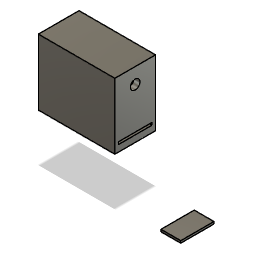
Kamera_arm-neu (Autodesk Fusion 360 design; units mm, degrees)
Autodesk Fusion 360 part; units mm, degrees
note: some values were not read from the file. Chosen so that the rebuilt part matches the saved one: which bodies a step acts on; which face or edge a step refers to. Set by a fixed rule: which sketch regions a step uses.
sketch "Skizze1" plane through (0, 0, 0) normal (0, 0, 1) x (1, 0, 0)
  line L0 (0, 0) -> (12, 0)
  line L1 (12, 0) -> (12, 24)
  line L2 (12, 24) -> (0, 24)
  line L3 (0, 24) -> (0, 0)
  dimension "d1" = 12
  dimension "d2" = 24
  constraint coincident L0.start L3.end
  constraint horizontal L0
  constraint perpendicular L0 L1
  constraint perpendicular L1 L2
  constraint perpendicular L0 L3
  measures "d1" distance of L0.start L0.end
  measures "d2" distance of L0.end L1.end
extrude "Extrusion1" add sketch "Skizze1" along normal blind 23 makes body 1
sketch "Skizze2" plane through (0, 0, 0) normal (0, 1, 0) x (1, 0, 0)
  line L0 (5, 5) -> (0.75, 5)
  circle A0 centre (2, 10.9) radius 1.5
  line L1 (0, 5.75) -> (0, 10)
  line L2 (0, 10) -> (0.8, 10)
  line L3 (0.8, 10) -> (0.8, 11.8)
  line L4 (0, 11.8) -> (0.8, 11.8)
  line L5 (0, 11.8) -> (0, 16.05)
  line L6 (0.75, 16.8) -> (5, 16.8)
  line L7 (5, 16.8) -> (5, 5)
  arc A1 (0, 5.75) -> (0.75, 5) centre (0.75, 5.75) ccw
  arc A2 (0.75, 16.8) -> (0, 16.05) centre (0.75, 16.05) ccw
  point P0 (0, 16.8)
  dimension "d7" = 3
  dimension "d9" = 5
  dimension "d10" = 0.75
  dimension "d11" = 0.75
  constraint horizontal L0
  constraint perpendicular L0 L1
  constraint coincident A0 L2.end
  constraint perpendicular L1 L2
  constraint coincident A0 L3.end
  constraint perpendicular L2 L3
  constraint perpendicular L3 L4
  constraint perpendicular L4 L5
  constraint perpendicular L5 L6
  constraint perpendicular L0 L7
  constraint tangent L0 A1
  constraint tangent L1 A1
  constraint coincident P0 L5
  constraint coincident P0 L6
  constraint tangent L5 A2
  constraint tangent L6 A2
  measures "d7" diameter of A0
  measures "d9" distance of L4.start P0
  measures "d10" radius of A1
  measures "d11" radius of A2
extrude "Extrusion2" add sketch "Skizze2" along normal blind 2.45 separate body contours L0 A0 L1 L2 L4 L5 L6 L7 A1 A2 makes body 2
move_body "Verschieben1" bodies 2 to x (1, 0, 0) y (0, 1, 0) z (0, 0, 1) at (0, 17.3532, -0.1472)
move_body "Verschieben2" bodies 2 to x (0, 0, 1) y (0, 1, 0) z (-1, 0, 0) at (-4.9472, 0, -4.9472)
copy_body "Körper kopieren/einfügen1" bodies 2 makes body 3
move_body "Verschieben3" bodies 3 to x (-1, 0, 0) y (0, 1, 0) z (0, 0, -1) at (12.15, 0, 25.1056)
move_body "Verschieben4" bodies 3 to x (1, 0, 0) y (0, 1, 0) z (0, 0, 1) at (0, 0, -2)
sketch "Skizze3" plane through (0, 0, 0) normal (0, 1, 0) x (1, 0, 0)
  circle A0 centre (25, -5) radius 6
  circle A1 centre (20, 9) radius 2.5
  circle A2 centre (31, -5) radius 2.75
  dimension "d14" = 12
  dimension "d15" = 5
  dimension "d16" = 5.5
  constraint coincident A0 A2.centre
  measures "d14" diameter of A0
  measures "d15" diameter of A1
  measures "d16" diameter of A2
extrude "Extrusion3" add sketch "Skizze3" along normal blind 2.5 separate body makes body 4 at (26.7719, 0, 5.8661) makes body 5 at (22.4969, 1.6667, -8.8754)
extrude "Extrusion4" add 1 faces at (26.6198, 2.5, 6.1216) along direction (0, 1, 0) blind 1.5 on bodies 4 bodies 4
move_body "Verschieben5" bodies 4 to x (1, 0, 0) y (0, 1, 0) z (0, 0, 1) at (0, 24, 0)
move_body "Verschieben6" bodies 4 to x (0, 0, 1) y (0, 1, 0) z (-1, 0, 0) at (10.9668, 0, -18.9668)
move_body "Verschieben7" bodies 5 to x (1, 0, 0) y (0, 1, 0) z (0, 0, 1) at (0, 28, 0)
move_body "Verschieben8" bodies 5 to x (1, 0, 0) y (0, 1, 0) z (0, 0, 1) at (-14, 0, 15)
combine "Kombinieren1" operation add target body 1 tool bodies 4
combine "Kombinieren2" operation add target body 5 tool bodies 1
combine "Kombinieren3" operation add target body 3 tool bodies 5 makes body 6 at (0, 8, 9.888)
combine "Kombinieren4" operation add target body 2 tool bodies 6
combine "Kombinieren5" operation add target body 2 tool bodies 3 makes body 7 at (10.468, 19.8032, 25.3466)
combine "Kombinieren6" operation add target body 7 tool bodies 2 makes body 8 at (0, 8, 9.888)
move_body "Verschieben9" bodies 7 to x (1, 0, 0) y (0, 1, 0) z (0, 0, 1) at (0, 0, -0.05)
move_body "Verschieben10" bodies 7 to x (1, 0, 0) y (0, 1, 0) z (0, 0, 1) at (0, 0, -0.05)
combine "Kombinieren7" operation add target body 7 tool bodies 8
move_body "Verschieben11" bodies 7 to x (1, 0, 0) y (0, 1, 0) z (0, 0, 1) at (0, 0, -28)
sketch "Skizze4" plane through (0, 0, 0) normal (0, 0, 1) x (1, 0, 0)
move_body "Verschieben12" bodies 7 to x (0, 0, -1) y (0, -1, 0) z (-1, 0, 0) at (0.1534, 30.5433, -0.1778)
sketch "Skizze5" plane through (0, 0, 0) normal (0, 0, 1) x (1, 0, 0)
  line L0 (55, 25) -> (105, 25)
  line L1 (105, 25) -> (105, 15)
  line L2 (55, -10) -> (55, 25)
  line L3 (55, -10) -> (105, 15)
  dimension "d21" = 50
  constraint horizontal L0
  constraint perpendicular L0 L1
  constraint perpendicular L0 L2
  measures "d21" distance of L0.start L0.end
extrude "Extrusion5" add sketch "Skizze5" along normal blind 20 separate body makes body 9
sketch "Skizze6" plane through (0, 0, 0) normal (0, 1, 0) x (1, 0, 0)
  circle A0 centre (125, -10) radius 2.5
  dimension "d24" = 5
  measures "d24" diameter of A0
hole "Bohrung1" at (95.1516, 25, 10.0122) direction (0, -1, 0) diameter 5 depth 2 tip angle 180 bodies 9
move_body "Verschieben13" bodies 9 to x (1, 0, 0) y (0, 1, 0) z (0, 0, 1) at (0, 0, -20)
sketch "Skizze7" plane through (0, 0, 0) normal (0, 0, 1) x (1, 0, 0)
  line L0 (125, 0) -> (131, 0)
  line L1 (131, 0) -> (131, 2.45)
  line L2 (164, 2.45) -> (164, 0)
  line L3 (164, 0) -> (170, 0)
  line L4 (170, 0) -> (170, 50)
  line L5 (170, 50) -> (125, 50)
  line L6 (125, 50) -> (125, 0)
  line L7 (131, 2.45) -> (136, 2.45)
  line L8 (136, 2.45) -> (136, 19.8)
  line L9 (164, 2.45) -> (159, 2.45)
  line L10 (159, 2.45) -> (159, 19.8)
  line L11 (136, 19.8) -> (159, 19.8)
  dimension "d31" = 2.45
  constraint horizontal L0
  constraint perpendicular L0 L1
  constraint perpendicular L2 L3
  constraint perpendicular L3 L4
  constraint perpendicular L4 L5
  constraint perpendicular L0 L6
  constraint perpendicular L1 L7
  constraint perpendicular L7 L8
  constraint perpendicular L2 L9
  constraint perpendicular L9 L10
  constraint perpendicular L10 L11
  measures "d31" distance of L0.end L1.end
extrude "Extrusion7" add sketch "Skizze7" against normal blind 30 separate body makes body 10
sketch "Skizze8" plane through (0, 0, 0) normal (0, 1, 0) x (1, 0, 0)
  line L0 (125, 40) -> (125, 49)
  line L1 (125, 49) -> (170, 49)
  line L2 (170, 49) -> (170, 40)
  line L3 (170, 40) -> (125, 40)
  line L4 (125, 55) -> (125, 64)
  line L5 (125, 64) -> (170, 64)
  line L6 (170, 64) -> (170, 55)
  line L7 (170, 55) -> (125, 55)
  constraint vertical L0
  constraint perpendicular L0 L1
  constraint perpendicular L1 L2
  constraint perpendicular L0 L3
  constraint perpendicular L1 L4
  constraint perpendicular L4 L5
  constraint perpendicular L1 L6
  constraint perpendicular L4 L7
extrude "Extrusion8" add sketch "Skizze8" along normal blind 20 separate body makes body 11 at (140, 13.3333, -49) makes body 12 at (140, 13.3333, -64)
move_body "Verschieben14" bodies 12 to x (1, 0, 0) y (0, 1, 0) z (0, 0, 1) at (0, 0, 55)
combine "Kombinieren8" operation add target body 10 tool bodies 12
move_body "Verschieben15" bodies 11 to x (1, 0, 0) y (0, 1, 0) z (0, 0, 1) at (0, 0, 19)
combine "Kombinieren9" operation add target body 10 tool bodies 11
copy_body "Körper kopieren/einfügen2" bodies 7 makes body 13
move_body "Verschieben16" bodies 13 to x (1, 0, 0) y (0, 1, 0) z (0, 0, 1) at (-40, 0, 0)
move_body "Verschieben17" bodies 10 to x (1, 0, 0) y (0, 1, 0) z (0, 0, 1) at (120, 0, 0)
move_body "Verschieben18" bodies 9 to x (1, 0, 0) y (0, 1, 0) z (0, 0, 1) at (-4.9193, 9.8387, -40)
copy_body "Körper kopieren/einfügen3" bodies 9 makes body 14
move_body "Verschieben19" bodies 14 to x (1, 0, 0) y (0, 1, 0) z (0, 0, 1) at (60, 0, 0)
copy_body "Körper kopieren/einfügen4" bodies 10 makes body 15
move_body "Verschieben20" bodies 15 to x (1, 0, 0) y (0, 1, 0) z (0, 0, 1) at (-70, 0, 0)
move_body "Verschieben21" bodies 9 14 to x (1, 0, 0) y (0, 1, 0) z (0, 0, 1) at (0, 0, 40)
move_body "Verschieben22" bodies 13 to x (1, 0, 0) y (0, 1, 0) z (0, 0, 1) at (0, -10.7, 0)
move_body "Verschieben23" bodies 13 to x (1, 0, 0) y (0, 1, 0) z (0, 0, 1) at (221, 0, -8.8)
move_body "Verschieben24" bodies 14 to x (1, 0, 0) y (0, 1, 0) z (0, 0, 1) at (53, -45, -5)
move_body "Verschieben25" bodies 13 15 14 to x (1, 0, 0) y (0, 1, 0) z (0, 0, 1) at (0, 45, 0)
sketch "Skizze9" plane through (0, 0, 0) normal (1, 0, 0) x (0, 0, -1)
  circle A0 centre (90, 40) radius 4
  dimension "d41" = 8
  measures "d41" diameter of A0
extrude "Extrusion9" add sketch "Skizze9" along normal blind 10 separate body makes body 16
move_body "Verschieben26" bodies 16 to x (0.965926, 0.258819, 0) y (-0.258819, 0.965926, 0) z (0, 0, 1) at (241.388, 43.4993, 74)
extrude "Extrusion10" add 1 faces at (230.7491, 83.2042, -13.7042) along direction (-0.965926, -0.258819, 0) blind 68 on bodies 16 bodies 15 16
extrude "Extrusion11" cut 1 faces at (165.0662, 65.6045, -13.7042) along direction (0.965926, 0.258819, 0) blind 67 on bodies 15 bodies 15 makes body 17 at (233.6627, 82.6339, -12.005)
move_body "Verschieben27" bodies 17 to x (1, 0, 0) y (0, 1, 0) z (0, 0, 1) at (1.9538, -7.2917, -57.0608)
extrude "Extrusion12" cut 1 faces at (242.3622, 78.5008, -70.7649) along direction (-0.965926, -0.258819, 0) blind 11 on bodies 17 bodies 17
sketch "Skizze10" plane through (0, 0, 0) normal (1, 0, 0) x (0, 0, -1)
  line L0 (-30, 10) -> (-20, 10)
  line L1 (-20, 10) -> (-20, 0)
  line L2 (-20, 0) -> (-30, 0)
  line L3 (-30, 0) -> (-30, 10)
  constraint horizontal L0
  constraint vertical L1
  constraint horizontal L2
  constraint vertical L3
extrude "Extrusion13" add sketch "Skizze10" along normal blind 2 bodies 17
sketch "Skizze11" plane through (0, 0, 0) normal (1, 0, 0) x (0, 0, -1)
  circle A0 centre (-25, 5) radius 2.5
  dimension "d52" = 5
  measures "d52" diameter of A0
extrude "Extrusion14" add sketch "Skizze11" against normal blind 2 bodies 17
move_body "Verschieben28" bodies 17 to x (-1, 0, 0) y (0, 1, 0) z (0, 0, -1) at (2, 0, 50)
move_body "Verschieben29" bodies 17 to x (1, 0, 0) y (0, 1, 0) z (0, 0, 1) at (220, 74, -41)
combine "Kombinieren10" operation add target body 15 tool bodies 17
move_body "Verschieben30" bodies 10 to x (1, 0, 0) y (0, 1, 0) z (0, 0, 1) at (-165, 45, 0)
move_body "Verschieben31" bodies 7 to x (1, 0, 0) y (0, 1, 0) z (0, 0, 1) at (86, 34.25, -9)
move_body "Verschieben32" bodies 9 to x (1, 0, 0) y (0, 1, 0) z (0, 0, 1) at (18, 0, -5)
move_body "Verschieben33" bodies 10 7 9 to x (1, 0, 0) y (0, 1, 0) z (0, 0, 1) at (-70, 0, 0)
sketch "Skizze12" plane through (0, 0, 0) normal (1, 0, 0) x (0, 0, -1)
  line L0 (50, 0) -> (78, 0)
  line L1 (78, 0) -> (78, 40)
  line L2 (50, 0) -> (50, 40)
  line L3 (50, 40) -> (78, 40)
  circle A0 centre (64, 32) radius 3.5
  dimension "d55" = 28
  dimension "d56" = 40
  dimension "d57" = 7
  constraint horizontal L0
  constraint perpendicular L0 L1
  constraint perpendicular L0 L2
  constraint perpendicular L1 L3
  measures "d55" distance of L0.start L0.end
  measures "d56" distance of L0.end L1.end
  measures "d57" diameter of A0
extrude "Extrusion15" add sketch "Skizze12" along normal blind 15 separate body contours L0 L1 L2 L3 | A0 makes body 18
sketch "Skizze13" plane through (0, 0, 0) normal (1, 0, 0) x (0, 0, -1)
  circle A0 centre (63.6687, 29.708) radius 3.5
  dimension "d60" = 7
  measures "d60" diameter of A0
extrude "Extrusion16" add sketch "Skizze13" against normal blind 3 bodies 18
move_body "Verschieben34" bodies 18 to x (-1, 0, 0) y (0, 1, 0) z (0, 0, -1) at (-6, 0, -156)
move_body "Verschieben35" bodies 18 to x (1, 0, 0) y (0, 1, 0) z (0, 0, 1) at (70, 0, 0)
extrude "Extrusion17" add 1 faces at (55, 78.3333, -10) along direction (1, 0, 0) blind 10 on bodies 10 bodies 10
move_body "Verschieben36" bodies 18 to x (1, 0, 0) y (0, 1, 0) z (0, 0, 1) at (0, 0, 77)
move_body "Verschieben37" bodies 18 to x (1, 0, 0) y (0, 1, 0) z (0, 0, 1) at (1, 0, 0)
extrude "Extrusion18" add 1 faces at (65, 78.3333, -10) along direction (1, 0, 0) blind 0.5 on bodies 10 bodies 10
extrude "Extrusion19" add 1 faces at (65.5, 78.3333, -10) along direction (1, 0, 0) blind 0.5 on bodies 10 bodies 10
extrude "Extrusion20" add 1 faces at (55, 40, -19.6667) along direction (0, 1, 0) blind 50 on bodies 18 bodies 10 18
extrude "Extrusion21" cut 1 faces at (55, 0, -19.6667) along direction (0, 1, 0) blind 90 on bodies 10 bodies 10 makes body 19 at (67, 29.5335, -11.8356)
extrude "Extrusion22" cut 1 faces at (68, 29.5341, -14.2552) along direction (-1, 0, 0) blind 3 on bodies 19 bodies 19
sketch "Skizze14" plane through (0, 0, 0) normal (1, 0, 0) x (0, 0, -1)
  line L0 (45, 5) -> (73, 5)
  line L1 (73, 5) -> (73, 7)
  line L2 (73, 7) -> (45, 7)
  line L3 (45, 7) -> (45, 5)
  constraint horizontal L0
  constraint vertical L1
  constraint horizontal L2
  constraint vertical L3
extrude "Extrusion23" add sketch "Skizze14" along normal blind 1 bodies 19
move_body "Verschieben38" bodies 19 to x (1, 0, 0) y (0, 1, 0) z (0, 0, 1) at (67, 0, 44)
move_body "Verschieben39" bodies 19 to x (1, 0, 0) y (0, 1, 0) z (0, 0, 1) at (0, 40.5, 0)
extrude "Extrusion24" add 1 faces at (67, 46.8333, -10.3333) along direction (-1, 0, 0) blind 17 on bodies 19 bodies 10 19
extrude "Extrusion25" cut 1 faces at (68, 46.8333, -10.3333) along direction (-1, 0, 0) blind 18.5 on bodies 10 bodies 10
sketch "Skizze15" plane through (0, 0, 0) normal (1, 0, 0) x (0, 0, -1)
  line L0 (40, 0) -> (67.8, 0)
  line L1 (40, 0) -> (40, 1.8)
  line L2 (40, 1.8) -> (67.8, 1.8)
  line L3 (67.8, 0) -> (67.8, 1.8)
  dimension "d81" = 27.8
  dimension "d82" = 1.8
  dimension "d83" = 27.8
  constraint horizontal L0
  constraint perpendicular L0 L1
  constraint perpendicular L1 L2
  measures "d81" distance of L0.start L0.end
  measures "d82" distance of L0.start L1.end
  measures "d83" distance of L1.end L2.end
extrude "Extrusion26" add sketch "Skizze15" along normal blind 16.5 separate body makes body 20
move_body "Verschieben40" bodies 20 to x (1, 0, 0) y (0, 1, 0) z (0, 0, 1) at (49.5, 45.5, 38.9)
sketch "Skizze16" plane through (0, 0, 0) normal (1, 0, 0) x (0, 0, -1)
  circle A0 centre (80, 20) radius 3
  dimension "d86" = 6
  measures "d86" diameter of A0
extrude "Extrusion27" add sketch "Skizze16" along normal blind 2 separate body makes body 21
move_body "Verschieben41" bodies 21 to x (1, 0, 0) y (0, 1, 0) z (0, 0, 1) at (75, 62, 65)
extrude "Extrusion28" add 1 faces at (75, 81.134, -14.5) along direction (-1, 0, 0) blind 18 on bodies 21 bodies 10 20 21
extrude "Extrusion29" cut 1 faces at (77, 81.134, -14.5) along direction (-1, 0, 0) blind 15 on bodies 10 bodies 10 makes body 22 at (58.6667, 83.0261, -17.8191)
extrude "Extrusion30" cut 1 faces at (62, 81.134, -14.5) along direction (-1, 0, 0) blind 5 on bodies 22 bodies 22
move_body "Verschieben42" bodies 20 to x (1, 0, 0) y (0, 1, 0) z (0, 0, 1) at (60, -45.5, 0)
extrude "Extrusion31" add 1 faces at (66, 58.0028, -15.0747) along direction (1, 0, 0) blind 8 on bodies 10 bodies 10 22
extrude "Extrusion32" cut 1 faces at (65, 58.0028, -14.9253) along direction (1, 0, 0) blind 4 on bodies 10 bodies 10
extrude "Extrusion33" cut 1 faces at (65, 45.3333, -19.6667) along direction (1, 0, 0) blind 3 on bodies 10 bodies 10
extrude "Extrusion34" add 3 faces at (67.6667, 61.6667, -30) (28.6667, 84.9333, -30) (28.6667, 53.2333, -30) along direction (0, 0, -1) blind 2 on bodies 10 bodies 10
extrude "Extrusion35" add 3 faces at (67.6667, 61.6667, 0) (28.6667, 84.9333, 0) (36.3333, 53.2333, 0) along direction (0, 0, 1) blind 2 on bodies 10 bodies 10
extrude "Extrusion36" add 1 faces at (14.7473, 19.8387, -25) along direction (0, 0, -1) blind 7 on bodies 9 bodies 9
extrude "Extrusion37" add 1 faces at (14.7473, 19.8387, -5) along direction (0, 0, 1) blind 7 on bodies 9 bodies 9
hole "Bohrung2" at (74, 82, -15) direction (-1, 0, 0) diameter 8 depth 10 tip angle 180 bodies 10
extrude "Extrusion38" add 1 faces at (38, 45, -5.3333) along direction (0, -1, 0) blind 5 on bodies 10 bodies 10
extrude "Extrusion39" add 1 faces at (28.6667, 64.8, -13) along direction (0, -1, 0) blind 5 on bodies 10 bodies 10
extrude "Extrusion40" add 1 faces at (47.3333, 47.45, -13) along direction (0, -1, 0) blind 5 on bodies 10 bodies 10
extrude "Extrusion41" add 1 faces at (19.3333, 47.45, -13) along direction (0, -1, 0) blind 5 on bodies 10 bodies 10
move_body "Verschieben43" bodies 7 to x (1, 0, 0) y (0, 1, 0) z (0, 0, 1) at (0, -5, 0)
sketch "Skizze17" plane through (0, 0, 0) normal (0, 1, 0) x (1, 0, 0)
  line L0 (16, 11) -> (13, 11)
  line L1 (16, 18) -> (13, 18)
  line L2 (13, 18) -> (13, 11)
  line L3 (16, 11) -> (21, 11)
  line L4 (21, 11) -> (21, 18)
  line L5 (21, 18) -> (16, 18)
  constraint perpendicular L1 L2
  constraint parallel L0 L3
  constraint perpendicular L3 L4
  constraint perpendicular L4 L5
extrude "Extrusion42" cut sketch "Skizze17" along normal blind 60 bodies 10
hidden bodies 9 13 14 15
